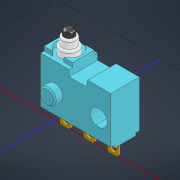
# Autodesk Inventor part: Microswitch Panasonic
Saved by Autodesk Inventor 2022.2 (Build 262287010, 287A)
## iProperties
Created: 2022-03-17
Part Number: Microswitch Panasonic
Material: PVC, hart
Document SubType Name: Modeling
Designer: sleib
Density: 1.29 g/cm^3
Appearance: Glatt - Weiß
Author: sleib
Autodesk Inventor part; units mm, degrees
ref_plane "YZ Plane" through (0, 0, 0) normal (1, 0, 0) x (0, 1, 0)
ref_plane "XZ Plane" through (0, 0, 0) normal (0, 1, 0) x (-1, 0, 0)
ref_plane "XY Plane" through (0, 0, 0) normal (0, 0, 1) x (1, 0, 0)
sketch "Skizze1" plane through (0, 0, 0) normal (0, 0, 1) x (1, 0, 0)
  line L0 (0, 0) -> (13.3, 0)
  line L1 (13.3, 0) -> (13.3, 8.8)
  line L2 (13.3, 8.8) -> (0, 8.8)
  line L3 (0, 8.8) -> (0, 0)
  circle A0 centre (2.7, 3.7) radius 1.5
  line L4 (0, 3.7) -> (13.3, 3.7) construction
  line L5 (10.4432, 5.2) -> (11.5568, 5.2)
  line L6 (10.4432, 2.2) -> (11.5568, 2.2)
  arc A1 (10.4432, 5.2) -> (10.4432, 2.2) centre (11, 3.7) ccw
  arc A2 (11.5568, 2.2) -> (11.5568, 5.2) centre (11, 3.7) ccw
  circle A3 centre (11, 3.7) radius 1.6 construction
  line L7 (1.12, 0) -> (3.12, 0)
  line L8 (3.12, 0) -> (3.12, -3.5)
  line L9 (3.12, -3.5) -> (1.12, -3.5)
  line L10 (1.12, -3.5) -> (1.12, 0)
  line L11 (5.65, 0) -> (7.65, 0)
  line L12 (7.65, 0) -> (7.65, -3.5)
  line L13 (7.65, -3.5) -> (5.65, -3.5)
  line L14 (5.65, -3.5) -> (5.65, 0)
  line L15 (10.18, 0) -> (12.18, 0)
  line L16 (12.18, 0) -> (12.18, -3.5)
  line L17 (12.18, -3.5) -> (10.18, -3.5)
  line L18 (10.18, -3.5) -> (10.18, 0)
  line L19 (0, 0) -> (0.25, 0)
  line L20 (0.25, 0) -> (0.25, -0.5)
  line L21 (0.25, -0.5) -> (0, -0.5)
  line L22 (0, -0.5) -> (0, 0)
  line L23 (13.3, 0) -> (13.05, 0)
  line L24 (13.05, 0) -> (13.05, -0.5)
  line L25 (13.05, -0.5) -> (13.3, -0.5)
  line L26 (13.3, -0.5) -> (13.3, 0)
  line L27 (2.12, 0) -> (2.12, -3.5) construction
  line L28 (6.65, 0) -> (6.65, -3.5) construction
  line L29 (11.18, 0) -> (11.18, -3.5) construction
  line L30 (11.18, -1.6) -> (11.18, -3.1) construction
  line L31 (10.58, -2.2) -> (10.58, -2.5)
  line L32 (11.78, -2.5) -> (11.78, -2.2)
  arc A4 (11.78, -2.2) -> (10.58, -2.2) centre (11.18, -2.2) ccw
  arc A5 (10.58, -2.5) -> (11.78, -2.5) centre (11.18, -2.5) ccw
  line L33 (2.12, -1.6) -> (2.12, -3.1) construction
  line L34 (1.52, -2.2) -> (1.52, -2.5)
  line L35 (2.72, -2.5) -> (2.72, -2.2)
  arc A6 (2.72, -2.2) -> (1.52, -2.2) centre (2.12, -2.2) ccw
  arc A7 (1.52, -2.5) -> (2.72, -2.5) centre (2.12, -2.5) ccw
  line L36 (6.65, -1.6) -> (6.65, -3.1) construction
  line L37 (6.05, -2.2) -> (6.05, -2.5)
  line L38 (7.25, -2.5) -> (7.25, -2.2)
  arc A8 (7.25, -2.2) -> (6.05, -2.2) centre (6.65, -2.2) ccw
  arc A9 (6.05, -2.5) -> (7.25, -2.5) centre (6.65, -2.5) ccw
  line L39 (5.4, 8.8) -> (5.4, 7.6)
  line L40 (5.4, 7.6) -> (8.7, 7.6)
  line L41 (8.7, 7.6) -> (8.9, 8.8)
  point P0 (13.175, -0.5)
  point P1 (11.18, -2.35)
  point P2 (2.12, -2.35)
  point P3 (6.65, -2.35)
  dimension "d0" = 13.3
  dimension "d3" = 3
  dimension "d4" = 3.7
  dimension "d5" = 5.1
  dimension "d6" = 3
  dimension "d7" = 2.7
  dimension "d8" = 8.3
  dimension "d10" = 3.2
  dimension "d11" = 4.2
  dimension "d12" = 0.25
  dimension "d13" = 0.25
  dimension "d14" = 4.53
  dimension "d15" = 4.53
  dimension "d16" = 2
  dimension "d17" = 3
  dimension "d18" = 1.5
  dimension "d19" = 1.2
  dimension "d23" = 1.5
  dimension "d24" = 1.2
  dimension "d25" = 0.4
  dimension "d26" = 0.4
  dimension "d27" = 1.5
  dimension "d28" = 1.2
  dimension "d29" = 0.4
  dimension "d30" = 5.4
  dimension "d32" = 3.3
  dimension "d33" = 1.2
  dimension "d34" = 3.5
  constraints: 90 end point, 22 point on circle, 22 point on line, 16 parallel, 14 tangent, 11 midpoint, 10 centre point, 8 horizontal, 7 perpendicular, 4 collinear, 1 coincident, 1 vertical, 1 other
  measures "d0" distance of L1.end L2.end
  measures "d3" diameter of A0
  measures "d4" distance between parallel lines of L0 L4
  measures "d5" distance between parallel lines of L2 L4
  measures "d6" distance between parallel lines of L6 L5
  measures "d7" distance from line of A0.centre L3
  measures "d8" distance of A1.centre A0.centre
  measures "d10" diameter of A3
  measures "d11" distance from line of point (13.175, -0.5) L4
  measures "d12" distance between parallel lines of L20 L22
  measures "d13" distance between parallel lines of L26 L24
  measures "d14" distance between parallel lines of L28 L27
  measures "d15" distance between parallel lines of L29 L28
  measures "d16" distance between parallel lines of L16 L18
  measures "d17" distance between parallel lines of L17 L25
  measures "d18" distance of L30.start L30.end
  measures "d19" diameter of A5
  measures "d23" distance of L33.start L33.end
  measures "d24" diameter of A7
  measures "d25" distance edge to line of A5 L17
  measures "d26" distance edge to line of A7 L9
  measures "d27" distance of L36.start L36.end
  measures "d28" diameter of A9
  measures "d29" distance edge to line of A9 L13
  measures "d30" distance from line of L39.start L3
  measures "d32" distance of L39.end L40.end
  measures "d33" distance of L39.start L39.end
  measures "d34" distance from line of L41.end L39
extrude "Extrusion1" add sketch "Skizze1" along normal mid plane 5.4 contours L3 L2 L39 L40 L41 L1 L0
extrude "Extrusion2" add sketch "Skizze1" along normal mid plane 8.4 contours A0
extrude "Extrusion3" add sketch "Skizze1" along normal mid plane 0.4 contours L0 L8 L9 L10 | L0 L12 L13 L14 | L0 L16 L17 L18
extrude "Extrusion4" add sketch "Skizze1" along normal mid plane 4.1 contours L0 L20 L21 L22 | L26 L25 L24 L0
chamfer "Fase1" distance 0.25 angle 45 2 edges at (1.2, 3.7, 4.2) (1.2, 3.7, -4.2)
chamfer "Fase2" distance 0.25 angle 45 6 edges at (12.18, -3.5, 0) (10.18, -3.5, 0) (7.65, -3.5, 0) (5.65, -3.5, 0) (3.12, -3.5, 0) (1.12, -3.5, 0)
sketch "Skizze2" plane through (0, 8.8, 2.7) normal (0, 1, 0) x (1, 0, 0)
  line L0 (0, 5.4) -> (0, 0) projected
  line L1 (5.4, 0) -> (0, 0) projected
  line L2 (5.4, 5.4) -> (5.4, 0) projected
  line L3 (0, 5.4) -> (5.4, 5.4) projected
  circle A0 centre (2.7, 2.7) radius 2.7 construction
  circle A1 centre (2.7, 2.7) radius 1.7
  circle A2 centre (2.7, 2.7) radius 1.3
  circle A3 centre (2.7, 2.7) radius 0.95
  line L4 (5.4, 5.4) -> (5.4, 0) projected
  line L5 (0, 4.75) -> (5.4, 4.75)
  line L6 (5.4, 4.75) -> (5.4, 0.65)
  line L7 (5.4, 0.65) -> (0, 0.65)
  line L8 (0, 0.65) -> (0, 4.75)
  line L9 (0, 4.75) -> (5.4, 0.65) construction
  line L10 (5.4, 4.75) -> (0, 0.65) construction
  circle A4 centre (2.7, 2.7) radius 2.3
  point P0 (0, 2.7)
  point P1 (3.7428, 4.75)
  point P2 (3.7428, 0.65)
  point P3 (5.4, 0.65)
  point P4 (1.6572, 0.65)
  point P5 (1.6572, 4.75)
  dimension "d49" = 1.9
  dimension "d50" = 2.6
  dimension "d51" = 3.4
  dimension "d61" = 4.1
  dimension "d62" = 4.6
  constraints: 12 end point, 5 centre point, 4 coincident, 3 tangent, 2 midpoint, 2 parallel, 1 horizontal, 1 perpendicular, 1 point on line
  measures "d49" diameter of A3
  measures "d50" diameter of A2
  measures "d51" diameter of A1
  measures "d61" distance of L5.end L6.end
  measures "d62" diameter of A4
extrude "Extrusion5" add sketch "Skizze2" along normal blind 4.1 contours A3
extrude "Extrusion6" add sketch "Skizze2" along normal blind 3 contours A2
extrude "Extrusion7" add sketch "Skizze2" along normal blind 1.5 contours A1
fillet "Rundung1" radius 0.5 1 edges at (1.75, 12.9, 0)
fillet "Rundung2" radius 0.4 1 edges at (1, 10.3, 0)
fillet "Rundung3" radius 0.35 1 edges at (1.4, 11.8, 0)
extrude "Extrusion8" add sketch "Skizze2" along normal blind 0.8 contours L5 A4 L7 L0 | L2 L7 A4 L5
